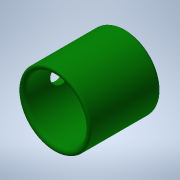
# Autodesk Inventor part: BUCHA
Saved by Autodesk Inventor 2021 (Build 250183000, 183)
## iProperties
Created: 2016-02-21
Part Number: BUCHA
Material: Genérico
Document SubType Name: Modeling
Designer: Everton
Density: 1 g/cm^3
Appearance: Padrão
Author: Everton
Autodesk Inventor part; units mm, degrees
ref_plane "YZ Plane" through (0, 0, 0) normal (1, 0, 0) x (0, 1, 0)
ref_plane "XZ Plane" through (0, 0, 0) normal (0, 1, 0) x (-1, 0, 0)
ref_plane "XY Plane" through (0, 0, 0) normal (0, 0, 1) x (1, 0, 0)
sketch "Sketch1" plane through (0, 0, 0) normal (0, 1, 0) x (-1, 0, 0)
  circle A0 centre (7.9604, -12.1069) radius 19
  circle A1 centre (7.9604, -12.1069) radius 16
  point P0 (0, 0)
  dimension "d0" = 38
  dimension "d1" = 32
  constraints: 2 centre point, 1 coincident
  measures "d0" diameter of A0
  measures "d1" diameter of A1
extrude "Extrusion1" add sketch "Sketch1" along normal blind 38
fillet "Fillet1" radius 2 2 edges at (11.0396, 38, -12.1069) (8.0396, 38, -12.1069)
fillet "Fillet2" radius 1 1 edges at (11.0396, 0, -12.1069)
fillet "Fillet3" radius 2 1 edges at (8.0396, 0, -12.1069)
sketch "Sketch2" plane through (0, 0, 0) normal (1, 0, 0) x (0, 1, 0)
  line L0 (39.783, 8.7002) -> (-1.9245, -33.003)
  circle A0 centre (18.9293, -12.1514) radius 5
  point P0 (0, 0)
  dimension "d7" = 10
  constraints: 2 end point, 1 centre point, 1 midpoint
  measures "d7" diameter of A0
extrude "Extrusion2" cut sketch "Sketch2" against normal blind 38
body "Solid1"
